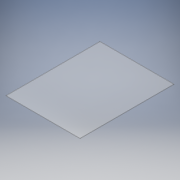
# Autodesk Inventor part: Small Wall
Saved by Autodesk Inventor 2017 (Build 210142000, 142)
## iProperties
Created: 2020-02-08
Part Number: Small Wall
Material: Polycarbonate, Clear
Document SubType Name: Modeling
Designer: S347041956
Density: 1.2 g/cm^3
Appearance: Polycarbonate - Clear
Author: S347041956
Autodesk Inventor part; units mm, degrees
ref_plane "YZ Plane" through (0, 0, 0) normal (1, 0, 0) x (0, 1, 0)
ref_plane "XZ Plane" through (0, 0, 0) normal (0, 1, 0) x (-1, 0, 0)
ref_plane "XY Plane" through (0, 0, 0) normal (0, 0, 1) x (1, 0, 0)
sketch "Sketch1" plane through (0, 0, 0) normal (1, 0, 0) x (0, 1, 0)
  line L0 (1.2792, 416.4647) -> (-1.2608, 416.4647)
  line L1 (-1.2608, 416.4647) -> (-1.2608, -2.6353)
  line L2 (-1.2608, -2.6353) -> (1.2792, -2.6353)
  line L3 (1.2792, -2.6353) -> (1.2792, 416.4647)
  point P0 (0, 0)
  dimension "d0" = 2.54
  dimension "d1" = 419.1
  constraints: 8 end point, 2 parallel, 1 horizontal, 1 perpendicular
  measures "d0" distance between parallel lines of L1 L3
  measures "d1" distance between parallel lines of L2 L0
extrude "Extrusion1" add sketch "Sketch1" along normal blind 330.2
body "Solid1"
